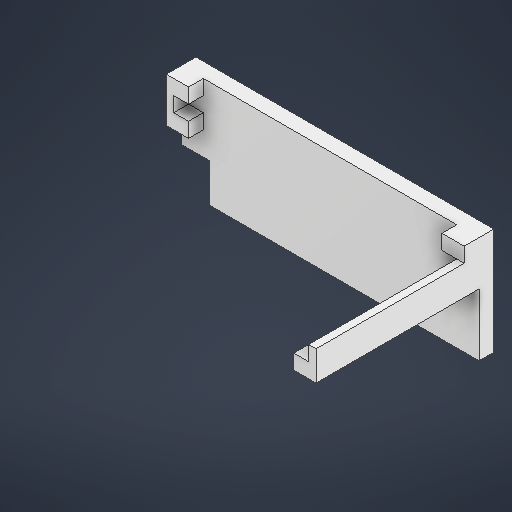
# Autodesk Inventor part: clip_zs042-command
Saved by Autodesk Inventor 2025.4 (Build 294407000, 407)
## iProperties
Created: 2026-01-02
Part Number: clip_zs042-command
Material: PC/ABS Plastic
Document SubType Name: Modeling
Designer: sam
Density: 1.1 g/cm^3
Appearance: Smooth - White
Author: sam
Autodesk Inventor part; units mm, degrees
ref_plane "YZ Plane" through (0, 0, 0) normal (1, 0, 0) x (0, 1, 0)
ref_plane "XZ Plane" through (0, 0, 0) normal (0, 1, 0) x (-1, 0, 0)
ref_plane "XY Plane" through (0, 0, 0) normal (0, 0, 1) x (1, 0, 0)
sketch "Sketch1" plane through (0, 0, 0) normal (0, 0, 1) x (1, 0, 0)
  line L0 (20.1, 7.2) -> (-20.1, 7.2)
  line L1 (-20.1, 7.2) -> (-20.1, -7.2)
  line L2 (-20.1, -7.2) -> (20.1, -7.2)
  line L3 (20.1, -7.2) -> (20.1, 7.2)
  line L4 (20.1, 7.2) -> (-20.1, -7.2) construction
  line L5 (-20.1, 7.2) -> (20.1, -7.2) construction
  line L6 (-20.1, -7.2) -> (-16.3, -7.2)
  line L7 (-16.3, -7.2) -> (-16.3, -2)
  line L8 (-16.3, -2) -> (-20.1, -2)
  line L9 (-20.1, -2) -> (-20.1, -7.2)
  point P0 (0, 0)
  point P1 (-20.1, -2)
  point P2 (-16.3, -7.2)
  dimension "d0" = 40.2
  dimension "d1" = 14.4
  dimension "d3" = 5.2
  dimension "d20" = 36.4
  constraints: 20 end point, 4 parallel, 2 horizontal, 2 midpoint, 2 perpendicular
  measures "d0" distance of L2.end L1.end
  measures "d1" distance of L1.end L0.end
  measures "d3" distance of L7.end L6.end
  measures "d20" distance between parallel lines of L3 L7
extrude "Extrusion1" add sketch "Sketch1" along normal blind 2 contours L3 L2 L7 L8 L1 L0
sketch "Sketch2" plane through (0, 0, 2) normal (0, 0, 1) x (1, 0, 0)
  line L0 (-20.1, 7.2) -> (-20.1, -2) projected
  line L1 (-20.1, 7.2) -> (-17.1, 7.2)
  line L2 (-17.1, 7.2) -> (-17.1, 1.2)
  line L3 (-17.1, 1.2) -> (-20.1, 1.2)
  line L4 (-20.1, 1.2) -> (-20.1, 7.2)
  line L5 (20.1, -7.2) -> (20.1, 7.2) projected
  line L6 (20.1, 7.2) -> (17.1, 7.2)
  line L7 (17.1, 7.2) -> (17.1, 1.2)
  line L8 (17.1, 1.2) -> (20.1, 1.2)
  line L9 (20.1, 1.2) -> (20.1, 7.2)
  line L10 (-20.1, 1.2) -> (-17.1, 1.2)
  line L11 (-17.1, 1.2) -> (-17.1, 3.2)
  line L12 (-17.1, 3.2) -> (-20.1, 3.2)
  line L13 (-20.1, 3.2) -> (-20.1, 1.2)
  line L14 (-20.1, 7.2) -> (-17.1, 7.2)
  line L15 (-17.1, 7.2) -> (-17.1, 5.2)
  line L16 (-17.1, 5.2) -> (-20.1, 5.2)
  line L17 (-20.1, 5.2) -> (-20.1, 7.2)
  line L18 (-20.1, 5.2) -> (-19.1, 5.2)
  line L19 (-19.1, 5.2) -> (-19.1, 3.2)
  line L20 (-19.1, 3.2) -> (-20.1, 3.2)
  line L21 (-20.1, 3.2) -> (-20.1, 5.2)
  line L22 (20.1, 7.2) -> (17.1, 7.2)
  line L23 (17.1, 7.2) -> (17.1, 5.2)
  line L24 (17.1, 5.2) -> (20.1, 5.2)
  line L25 (20.1, 5.2) -> (20.1, 7.2)
  line L26 (17.1, 1.2) -> (20.1, 1.2)
  line L27 (20.1, 1.2) -> (20.1, 3.2)
  line L28 (20.1, 3.2) -> (17.1, 3.2)
  line L29 (17.1, 3.2) -> (17.1, 1.2)
  line L30 (20.1, 3.2) -> (19.1, 3.2)
  line L31 (19.1, 3.2) -> (19.1, 5.2)
  line L32 (19.1, 5.2) -> (20.1, 5.2)
  line L33 (20.1, 5.2) -> (20.1, 3.2)
  point P0 (0, 0)
  dimension "d6" = 3
  dimension "d7" = 6
  dimension "d8" = 3
  dimension "d9" = 6
  dimension "d10" = 2
  dimension "d11" = 2
  dimension "d12" = 1
  dimension "d13" = 2
  dimension "d14" = 2
  dimension "d15" = 1
  constraints: 64 end point, 16 parallel, 8 horizontal, 8 perpendicular, 6 point on line
  measures "d6" distance of L2.end L3.end
  measures "d7" distance of L1.end L2.end
  measures "d8" distance of L8.end L7.end
  measures "d9" distance of L7.end L6.end
  measures "d10" distance of L11.end L10.end
  measures "d11" distance of L14.end L15.end
  measures "d12" distance of L19.end L20.end
  measures "d13" distance of L23.end L22.end
  measures "d14" distance of L27.end L26.end
  measures "d15" distance of L31.end L32.end
extrude "Extrusion2" add sketch "Sketch2" along normal blind 2 contours L1 L2 L16 L0 | L16 L19 L12 L0 | L12 L2 L3 L0 | L8 L7 L28 L5 | L28 L31 L24 L5 | L24 L7 L6 L5
sketch "Sketch3" plane through (0, 0, 4) normal (0, 0, 1) x (1, 0, 0)
  line L0 (17.1, 3.2) -> (17.1, 1.2) projected
  line L1 (17.1, 1.2) -> (20.1, 1.2) projected
  line L2 (20.1, 1.2) -> (20.1, 7.2) projected
  line L3 (20.1, 7.2) -> (17.1, 7.2) projected
  line L4 (17.1, 7.2) -> (17.1, 5.2) projected
  line L5 (17.1, 5.2) -> (19.1, 5.2) projected
  line L6 (19.1, 5.2) -> (19.1, 3.2) projected
  line L7 (19.1, 3.2) -> (17.1, 3.2) projected
  line L8 (19.1, 5.2) -> (20.1, 5.2)
  point P0 (0, 0)
  constraints: 2 end point, 1 perpendicular, 1 point on line
extrude "Extrusion3" add sketch "Sketch3" along normal blind 20 contours L7 L6 L8 L2 L1 L0
body "Solid1"
